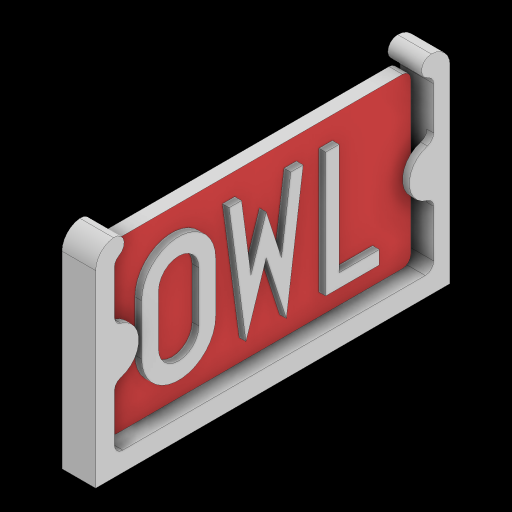
# Autodesk Inventor part: plate
Saved by Autodesk Inventor 2024.1 (Build 281209000, 209)
## iProperties
Created: 2025-05-12
Part Number: plate
Material: Generic
Document SubType Name: Modeling
Designer: Teddy
Density: 1 g/cm^3
Appearance: Default
Author: Teddy
Autodesk Inventor part; units mm, degrees
ref_plane "YZ Plane" through (0, 0, 0) normal (1, 0, 0) x (0, 1, 0)
ref_plane "XZ Plane" through (0, 0, 0) normal (0, 1, 0) x (-1, 0, 0)
ref_plane "XY Plane" through (0, 0, 0) normal (0, 0, 1) x (1, 0, 0)
sketch "Sketch1" plane through (0, 0, 0) normal (1, 0, 0) x (0, 1, 0)
  point P0 (0, 0)
sketch "Sketch2" plane through (0, 0, 0) normal (1, 0, 0) x (0, 1, 0)
  line L0 (-31.75, 57.15) -> (31.75, 57.15)
  line L1 (31.75, 57.15) -> (31.75, -57.15)
  line L2 (31.75, -57.15) -> (-31.75, -57.15)
  line L3 (-31.75, -57.15) -> (-31.75, 57.15)
  line L4 (-31.75, 57.15) -> (31.75, -57.15) construction
  line L5 (31.75, 57.15) -> (-31.75, -57.15) construction
  circle A0 centre (34.2977, 59.8004) radius 3.6763
  circle A1 centre (34.3401, -59.759) radius 3.6763
  line L6 (34.2977, 59.8004) -> (-33.2225, 59.8004)
  line L7 (-33.2225, 59.8004) -> (-33.2225, -60.6799)
  line L8 (-33.2225, -60.6799) -> (30.781, -60.6799)
  line L9 (34.2977, -63.4351) -> (-37.1507, -63.4351)
  line L10 (-37.1507, -63.4351) -> (-37.1507, 63.4768)
  line L11 (-37.1507, 63.4768) -> (34.2977, 63.4768)
  line L12 (30.5673, 66.8746) -> (-40.5486, 66.8746)
  line L13 (-40.5486, 66.8746) -> (-40.5486, -66.833)
  line L14 (-40.5486, -66.833) -> (30.9179, -66.833)
  arc A2 (37.958, 60.1427) -> (30.5673, 66.8746) centre (30.5673, 59.4517) ccw
  arc A3 (30.9179, -66.833) -> (38.0163, -59.7854) centre (30.9179, -59.7345) ccw
  point P0 (0, 0)
  point P1 (30.6213, 59.8004)
  dimension "d0" = 63.5
  dimension "d1" = 114.3
  constraints: 30 end point, 11 point on circle, 5 perpendicular, 5 tangent, 4 centre point, 3 parallel, 2 horizontal, 2 midpoint, 1 equal radius, 2 other
  measures "d0" distance between parallel lines of L3 L1
  measures "d1" distance between parallel lines of L0 L2
extrude "Extrusion1" add sketch "Sketch2" along normal blind 7.62 contours A0 | A1 | L6 L7 L8 A1 L9 L10 L11 A0 | A0 L11 L10 L9 A1 A3 L14 L13 L12 A2
fillet "Fillet1" radius 3.175 2 edges at (3.81, 30.781, -60.6799) (3.81, 30.6213, 59.8004)
sketch "Sketch3" plane through (7.62, 0, 0) normal (1, 0, 0) x (0, 0, -1)
  line L0 (-40.64, -9.525) -> (-40.64, 9.525)
  line L1 (-40.64, 9.525) -> (-25.4, 9.525) construction
  line L2 (-25.4, 9.525) -> (-25.4, -9.525)
  line L3 (-25.4, -9.525) -> (-40.64, -9.525) construction
  arc A0 (-40.64, -9.525) -> (-25.4, -9.525) centre (-33.02, -9.525) ccw
  arc A1 (-25.4, 9.525) -> (-40.64, 9.525) centre (-33.02, 9.525) ccw
  line L4 (-46.99, 9.525) -> (-46.99, -9.525)
  arc A2 (-46.99, -9.525) -> (-19.05, -9.525) centre (-33.02, -9.525) ccw
  line L5 (-19.05, -9.525) -> (-19.05, 9.525)
  arc A3 (-19.05, 9.525) -> (-46.99, 9.525) centre (-33.02, 9.525) ccw
  line L6 (-13.97, 23.4062) -> (-7.62, -23.495)
  line L7 (-7.62, -23.495) -> (0, 0)
  line L8 (0, 0) -> (7.6197, -23.5927)
  line L9 (7.6197, -23.5927) -> (13.97, 23.407)
  line L10 (-9.3882, 24.1126) -> (-5.7552, -2.7208)
  line L11 (-5.7552, -2.7208) -> (0.0092, 15.053)
  line L12 (0.0092, 15.053) -> (5.7587, -2.749)
  line L13 (5.7587, -2.749) -> (9.3883, 24.1143)
  line L14 (-13.97, 23.4062) -> (-9.2926, 23.4062)
  line L15 (13.97, 23.407) -> (9.2927, 23.4062)
  line L16 (22.4524, 23.3392) -> (22.4524, -23.6655)
  line L17 (22.4524, -23.6655) -> (42.7011, -23.6655)
  line L18 (42.7011, -23.6655) -> (42.7011, -18.5855)
  line L19 (42.7011, -18.5855) -> (27.5324, -18.5855)
  line L20 (27.5324, -18.5855) -> (27.5324, 23.3392)
  line L21 (27.5324, 23.3392) -> (22.4524, 23.3392)
  line L22 (-46.99, 0) -> (-59.8004, 0) construction
  line L23 (-59.8004, -33.2225) -> (-59.8004, 28.2264) construction
  line L24 (32.5768, -23.6655) -> (32.5768, -33.2225) construction
  line L25 (60.6799, -33.2225) -> (-59.8004, -33.2225) construction
  point P0 (-25.4, 0)
  dimension "d5" = 15.24
  dimension "d6" = 25.4
  dimension "d7" = 19.05
  dimension "d8" = 6.35
  dimension "d9" = 27.94
  dimension "d10" = 13.97
  dimension "d11" = 15.24
  dimension "d12" = 7.62
  dimension "d13" = 5.08
  dimension "d14" = 5.08
  constraints: 48 end point, 10 perpendicular, 8 point on circle, 5 midpoint, 5 point on line, 4 centre point, 4 tangent, 1 horizontal, 1 horizontal alignment, 1 parallel, 1 vertical, 6 other
  measures "d5" distance between parallel lines of L2 L0
  measures "d6" distance from line of L7.end L2
  measures "d7" distance of point (-33.02, -9.525) point (-33.02, 9.525)
  measures "d8" distance between parallel lines of L0 L4
  measures "d9" distance of L9.end L6.start
  measures "d10" horizontal distance of L7.end L6.start
  measures "d11" distance of L8.end L6.end
  measures "d12" horizontal distance of L7.end L6.end
  measures "d13" distance of L17.end L18.end
  measures "d14" distance between parallel lines of L20 L16
extrude "Extrusion2" add sketch "Sketch3" against normal blind 2.54 separate body
sketch "Sketch4" plane through (5.08, 0, 0) normal (-1, 0, 0) x (0, 0, 1)
  line L0 (-57.15, -31.75) -> (57.15, -31.75)
  line L1 (57.15, -31.75) -> (57.15, 31.75)
  line L2 (57.15, 31.75) -> (-57.15, 31.75)
  line L3 (-57.15, 31.75) -> (-57.15, -31.75)
  line L4 (-57.15, -31.75) -> (57.15, 31.75) construction
  line L5 (57.15, -31.75) -> (-57.15, 31.75) construction
  point P0 (0, 0)
  dimension "d17" = 114.3
  dimension "d18" = 63.5
  constraints: 12 end point, 2 midpoint, 2 parallel, 1 horizontal, 1 perpendicular
  measures "d17" distance of L2.end L1.end
  measures "d18" distance between parallel lines of L0 L2
extrude "Extrusion3" add sketch "Sketch4" along normal blind 5.08 bodies 2
fillet "Fillet2" radius 3.175 4 edges at (2.54, 31.75, -57.15) (2.54, 31.75, 57.15) (2.54, -31.75, 57.15) (2.54, -31.75, -57.15)
sketch "Sketch5" plane through (7.62, 0, 0) normal (1, 0, 0) x (0, 0, -1)
  line L0 (-59.8004, -33.2225) -> (-59.8004, 28.2264) projected
  arc A0 (-59.8004, -9.4214) -> (-59.8004, 8.9856) centre (-59.8004, -0.2179) ccw
  line L1 (-59.8004, -33.2225) -> (-59.8004, 28.2264) projected
  line L2 (60.6799, 27.8701) -> (60.6799, -33.2225) projected
  arc A1 (60.6799, 8.9979) -> (60.6799, -9.4337) centre (60.6799, -0.2179) ccw
  arc A2 (-60.1427, 37.958) -> (-66.8746, 30.5673) centre (-59.4517, 30.5673) ccw projected
  line L3 (-66.8746, 30.5673) -> (-66.8746, -40.5486) projected
  line L4 (-66.8746, -40.5486) -> (66.833, -40.5486) projected
  line L5 (66.833, -40.5486) -> (66.833, 30.9179) projected
  arc A3 (66.833, 30.9179) -> (59.7854, 38.0163) centre (59.7345, 30.9179) ccw projected
  arc A4 (59.7854, 38.0163) -> (58.5495, 30.8684) centre (59.759, 34.3401) ccw projected
  arc A5 (60.6799, 27.8701) -> (58.5495, 30.8684) centre (57.5049, 27.8701) ccw projected
  line L6 (60.6799, 27.8701) -> (60.6799, -33.2225) projected
  line L7 (60.6799, -33.2225) -> (-59.8004, -33.2225) projected
  line L8 (-59.8004, -33.2225) -> (-59.8004, 28.2264) projected
  arc A6 (-58.0968, 31.0399) -> (-59.8004, 28.2264) centre (-56.6254, 28.2264) ccw projected
  arc A7 (-58.0968, 31.0399) -> (-60.1427, 37.958) centre (-59.8004, 34.2977) ccw projected
  point P0 (0, 0)
  constraints: 6 point on line, 4 point on circle, 2 centre point
extrude "Extrusion4" add sketch "Sketch5" along normal blind 2.54 bodies 1
sketch "Sketch6" plane through (0, 0, 0) normal (-1, 0, 0) x (0, 0, 1)
  line L0 (-60.6799, 8.9979) -> (-60.6799, -9.4337) projected
  arc A0 (-60.6799, -9.4337) -> (-60.6799, 8.9979) centre (-60.6799, -0.2179) ccw projected
  line L1 (57.15, -28.575) -> (57.15, 28.575) projected
  line L2 (59.8004, -9.4214) -> (59.8004, 8.9856) projected
  arc A1 (59.8004, 8.9856) -> (59.8004, -9.4214) centre (59.8004, -0.2179) ccw projected
  arc A2 (66.8746, 30.5673) -> (60.1427, 37.958) centre (59.4517, 30.5673) ccw projected
  arc A3 (60.1427, 37.958) -> (58.0968, 31.0399) centre (59.8004, 34.2977) ccw projected
  arc A4 (59.8004, 28.2264) -> (58.0968, 31.0399) centre (56.6254, 28.2264) ccw projected
  line L3 (59.8004, -33.2225) -> (59.8004, 28.2264) projected
  line L4 (-60.6799, -33.2225) -> (59.8004, -33.2225) projected
  line L5 (-60.6799, 27.8701) -> (-60.6799, -33.2225) projected
  arc A5 (-58.5495, 30.8684) -> (-60.6799, 27.8701) centre (-57.5049, 27.8701) ccw projected
  arc A6 (-58.5495, 30.8684) -> (-59.7854, 38.0163) centre (-59.759, 34.3401) ccw projected
  arc A7 (-59.7854, 38.0163) -> (-66.833, 30.9179) centre (-59.7345, 30.9179) ccw projected
  line L6 (-66.833, -40.5486) -> (-66.833, 30.9179) projected
  line L7 (66.8746, -40.5486) -> (-66.833, -40.5486) projected
  line L8 (66.8746, 30.5673) -> (66.8746, -40.5486) projected
  point P0 (0, 0)
extrude "Extrusion5" add sketch "Sketch6" along normal blind 2.54 bodies 1
fillet "Fillet3" radius 3.175 8 edges at (-1.27, 8.9979, -60.6799) (-1.27, -9.4337, -60.6799) (-1.27, 8.9856, 59.8004) (-1.27, -9.4214, 59.8004) (8.89, 8.9979, -60.6799) (8.89, -9.4337, -60.6799) (8.89, 8.9856, 59.8004) (8.89, -9.4214, 59.8004)
fillet "Fillet4" radius 3.175 2 edges at (3.81, -33.2225, -60.6799) (3.81, -33.2225, 59.8004)
fillet "Fillet5" [suppressed]
body "Solid1"
body "Solid2"
